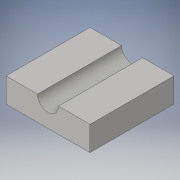
# Autodesk Inventor part: BottomOfSquareSupport
Saved by Autodesk Inventor 2016 SP1 (Build 200210100, 210)
## iProperties
Created: 2015-12-08
Part Number: BottomOfSquareSupport
Material: Generic
Document SubType Name: Modeling
Designer: steele
Density: 1 g/cm^3
Appearance: Default
Author: steele
Autodesk Inventor part; units mm, degrees
ref_plane "YZ Plane" through (0, 0, 0) normal (1, 0, 0) x (0, 1, 0)
ref_plane "XZ Plane" through (0, 0, 0) normal (0, 1, 0) x (-1, 0, 0)
ref_plane "XY Plane" through (0, 0, 0) normal (0, 0, 1) x (1, 0, 0)
sketch "Sketch1" plane through (0, 0, 0) normal (0, 1, 0) x (-1, 0, 0)
  line L0 (-19.05, 19.05) -> (-19.05, -19.05)
  line L1 (-19.05, -19.05) -> (19.05, -19.05)
  line L2 (19.05, -19.05) -> (19.05, 19.05)
  line L3 (19.05, 19.05) -> (-19.05, 19.05)
  line L4 (-19.05, 19.05) -> (19.05, -19.05) construction
  line L5 (-19.05, -19.05) -> (19.05, 19.05) construction
  point P0 (0, 0)
  dimension "d0" = 38.1
  constraints: 12 end point, 2 midpoint, 2 parallel, 2 perpendicular, 1 vertical
  measures "d0" distance of L0.start L0.end
extrude "Extrusion1" add sketch "Sketch1" along normal blind 11.1125
sketch "Sketch2" plane through (-19.05, 0, 19.05) normal (0, 0, 1) x (1, 0, 0)
  line L0 (38.1, 11.1125) -> (0, 11.1125) projected
  arc A0 (14.2875, 11.1125) -> (23.8125, 11.1125) centre (19.05, 11.1125) ccw
  point P0 (19.05, 0)
  dimension "d3" = 9.525
  constraints: 2 point on circle, 2 point on line, 1 centre point, 1 midpoint
  measures "d3" diameter of A0
extrude "Extrusion2" cut sketch "Sketch2" against normal through all
equation "\"d0\" = width"
equation "\"d1\" = heightOfBottomHole"
equation "\"d3\" = bottomHoleDiam"
equation "\"d4\" = deltaBottomToTop"
equation "\"bottomHoleDiam\" = 9.525"
equation "\"width\" = 38.1"
equation "\"height\" = deltaBottomToTop + heightOfBottomHole + heightOfTopHole"
equation "\"deltaBottomToTop\" = 25.4"
equation "\"heightOfBottomHole\" = 11.1125"
equation "\"heightOfTopHole\" = 11.1125"
body "Solid1"
